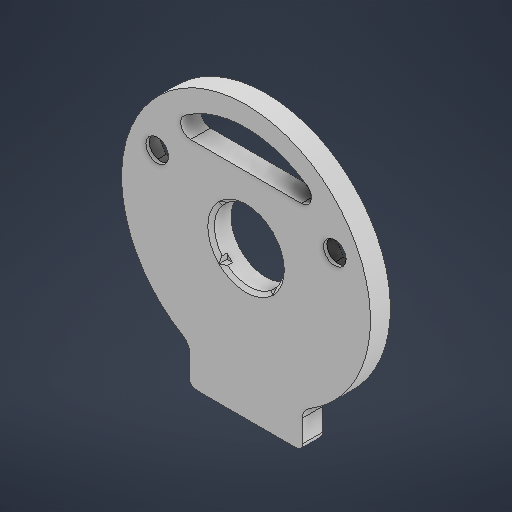
# Autodesk Inventor part: Držák-Cam+ir
Saved by Autodesk Inventor 2026 (Build 300175000, 175)
## iProperties
Created: 2025-06-20
Part Number: Držák-Cam+ir
Material: Všeobecné
Document SubType Name: Modeling
Designer: vadim
Density: 1 g/cm^3
Appearance: Výchozí
Author: vadim
Autodesk Inventor part; units mm, degrees
ref_plane "YZ Plane" through (0, 0, 0) normal (1, 0, 0) x (0, 1, 0)
ref_plane "XZ Plane" through (0, 0, 0) normal (0, 1, 0) x (-1, 0, 0)
ref_plane "XY Plane" through (0, 0, 0) normal (0, 0, 1) x (1, 0, 0)
sketch "Náčrt1" plane through (0, 0, 0) normal (0, 0, 1) x (1, 0, 0)
  circle A0 centre (0, 0) radius 5.25
  arc A1 (8.5, -16.6565) -> (-8.5, -16.6565) centre (0, 0) ccw
  line L0 (-13.35, 6.1) -> (13.35, 6.1)
  line L1 (0, 18.7) -> (0, -18.7)
  line L2 (8.5, -16.6565) -> (8.5, -22.2)
  line L3 (8.5, -22.2) -> (-8.5, -22.2)
  line L4 (-8.5, -22.2) -> (-8.5, -16.6565)
  line L5 (0, -18.7) -> (8.5, -22.2) construction
  line L6 (0, -18.7) -> (-8.5, -22.2) construction
  line L7 (-10.0014, 6.1) -> (-11.6757, 3.2)
  line L8 (-11.6757, 3.2) -> (-15.0243, 3.2)
  line L9 (-15.0243, 3.2) -> (-16.6986, 6.1)
  line L10 (-16.6986, 6.1) -> (-15.0243, 9)
  line L11 (-15.0243, 9) -> (-11.6757, 9)
  line L12 (-11.6757, 9) -> (-10.0014, 6.1)
  line L13 (16.6986, 6.1) -> (15.0243, 3.2)
  line L14 (15.0243, 3.2) -> (11.6757, 3.2)
  line L15 (11.6757, 3.2) -> (10.0014, 6.1)
  line L16 (10.0014, 6.1) -> (11.6757, 9)
  line L17 (11.6757, 9) -> (15.0243, 9)
  line L18 (15.0243, 9) -> (16.6986, 6.1)
  circle A2 centre (-13.35, 6.1) radius 1.7
  circle A3 centre (13.35, 6.1) radius 1.7
  line L19 (-12.1033, 10) -> (12.1033, 10)
  arc A4 (12.1033, 10) -> (-12.1033, 10) centre (0, 0) ccw
  line L20 (4.1, 4.1) -> (-4.1, 4.1)
  line L21 (-4.1, 4.1) -> (-4.1, -4.1)
  line L22 (-4.1, -4.1) -> (4.1, -4.1)
  line L23 (4.1, -4.1) -> (4.1, 4.1)
  line L24 (4.1, 4.1) -> (-4.1, -4.1) construction
  line L25 (-4.1, 4.1) -> (4.1, -4.1) construction
  point P0 (4.1, -3.2791)
  point P1 (3.2791, -4.1)
  point P2 (-3.2791, -4.1)
  point P3 (-4.1, -3.2791)
  point P4 (-4.1, 3.2791)
  point P5 (-3.2791, 4.1)
  point P6 (4.1, 3.2791)
  point P7 (3.2791, 4.1)
  dimension "d0" = 10.5
  dimension "d1" = 37.4
  dimension "d2" = 26.7
  dimension "d3" = 17
  dimension "d5" = 22.2
  dimension "d6" = 5.8
  dimension "d7" = 6.1
  dimension "d8" = 5.8
  dimension "d9" = 3.4
  dimension "d10" = 3.4
  dimension "d12" = 10
  dimension "d14" = 3
  dimension "d25" = 8.2
  dimension "d26" = 8.2
  constraints: 52 end point, 6 coincident, 5 centre point, 5 point on circle, 4 midpoint, 3 horizontal, 3 parallel, 2 perpendicular, 1 point on line, 1 symmetric about line, 1 vertical, 27 other
  measures "d0" diameter of A0
  measures "d1" diameter of A1
  measures "d2" distance of L0.start L0.end
  measures "d3" distance of L2.end L3.end
  measures "d5" distance from line of L3 point (0, 0)
  measures "d6" distance between parallel lines of L8 L11
  measures "d7" vertical distance of point (0, 0) L0.start
  measures "d8" distance between parallel lines of L14 L17
  measures "d9" diameter of A2
  measures "d10" diameter of A3
  measures "d12" distance from line of L19 A1.centre
  measures "d14" radial gap between concentric circles of A1 A4
  measures "d25" distance of L22.end L21.end
  measures "d26" distance of L21.end L20.end
extrude "Vysunutí1" add sketch "Náčrt1" along normal blind 0.5 contours A0 L20 L23 | L23 L22 A0 | A0 L21 L20 | L22 L21 A0 | L2 L3 L4 A1 | L7 L8 L9 L10 L11 L12 | L13 L14 L15 L16 L17 L18
extrude "Vysunutí2" add sketch "Náčrt1" against normal blind 2.5 contours A0 L20 L23 | L23 L22 A0 | A0 L21 L20 | L22 L21 A0 | L2 L3 L4 A1
fillet "Zaoblení1" radius 1.5 2 edges at (12.1033, 10, -1) (-12.1033, 10, -1)
fillet "Zaoblení2" radius 1 2 edges at (8.5, -22.2, -1) (-8.5, -22.2, -1)
fillet "Zaoblení3" radius 2 2 edges at (8.5, -16.6565, -1) (-8.5, -16.6565, -1)
chamfer "Zkosení1" distance 0.5 angle 45 1 edges at (-5.25, 0, 0.5)
extrude "Vysunutí3" cut sketch "Náčrt1" along normal blind 0.75 and the other way blind 0.75 contours A0 L20 L23 | L23 L22 A0 | A0 L21 L20 | L22 L21 A0
